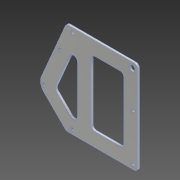
# Autodesk Inventor part: palmrest-plate
Saved by Autodesk Inventor 2018 (Build 220112000, 112)
## iProperties
Created: 2018-07-10
Part Number: palmrest-plate
Material: アルミニウム 6061
Document SubType Name: Sheet Metal
Designer: NaMACHAN
Mass: 31.1777 g
Surface Area: 131.125 cm^2
Volume: 11.5473 cm^3
Density: 2.7 g/cm^3
Sheet Metal Rule: Default
Appearance: アルミニウム - フラット
Flat Pattern Width: 10.477 cm
Flat Pattern Length: 10 cm
Flat Pattern Area: 104.77 cm^2
Sheet Metal Width: 104.770 mm
Sheet Metal Length: 100.000 mm
Sheet Metal Area: 10476.990 mm^2
Author: NaMACHAN
Autodesk Inventor part; units mm, degrees
ref_plane "YZ Plane" through (0, 0, 0) normal (1, 0, 0) x (0, 1, 0)
ref_plane "XZ Plane" through (0, 0, 0) normal (0, 1, 0) x (-1, 0, 0)
ref_plane "XY Plane" through (0, 0, 0) normal (0, 0, 1) x (1, 0, 0)
sketch "スケッチ4" plane through (0, 0, 0) normal (0, 1, 0) x (-1, 0, 0)
  line L0 (0, 0) -> (0, -100)
  line L1 (0, -100) -> (77, -100)
  line L2 (77, -100) -> (107, -70)
  line L3 (107, -70) -> (77, 0)
  line L4 (77, 0) -> (0, 0)
  line L5 (89.2124, -66.5744) -> (70.7868, -85)
  line L6 (65, -85) -> (65, -15)
  line L7 (67.1091, -15) -> (89.2124, -66.5744)
  line L8 (50, -85) -> (50, -15)
  line L9 (50, -15) -> (15, -15)
  line L10 (15, -15) -> (15, -85)
  line L11 (15, -85) -> (50, -85)
  line L12 (70.7868, -85) -> (65, -85)
  line L13 (67.1091, -15) -> (65, -15)
  dimension "d21" = 77
  dimension "d22" = 100
  dimension "d24" = 30
  dimension "d25" = 30
  dimension "d52" = 15
  dimension "d54" = 15
  dimension "d55" = 15
  dimension "d56" = 50
  dimension "d57" = 15
  dimension "d58" = 15
  dimension "d59" = 15
  measures "d21" distance of L3.end L0.start
  measures "d22" distance of L0.start L0.end
  measures "d24" horizontal distance of L1.end L2.end
  measures "d25" horizontal distance of L3.end L2.end
  measures "d52" distance between parallel lines of L0 L10
  measures "d54" distance between parallel lines of L4 L9
  measures "d55" distance between parallel lines of L1 L11
  measures "d56" distance between parallel lines of L0 L8
  measures "d57" distance between parallel lines of L8 L6
  measures "d58" distance between parallel lines of L3 L7
  measures "d59" distance between parallel lines of L2 L5
extrude "プレート2" add sketch "スケッチ4" along normal blind 2
fillet "コーナーR3" radius 12 1 edges at (-107, 1, -70)
fillet "コーナーR4" radius 4 4 edges at (-77, 1, -100) (0, 1, -100) (0, 1, 0) (-77, 1, 0)
sketch "スケッチ5" plane through (0, 2, 0) normal (0, 1, 0) x (1, 0, 0)
  line L0 (-4, 0) -> (-74.3624, 0) projected
  line L1 (0, 96) -> (0, 4) projected
  line L2 (-75.3431, 100) -> (-4, 100) projected
  point P0 (0, 0)
  point P1 (-70, 5)
  point P2 (-70, 95)
  point P3 (-5, 95)
  point P4 (-5, 5)
  point P5 (-5, 45)
  dimension "d29" = 5
  dimension "d30" = 5
  dimension "d31" = 5
  dimension "d40" = 65
  dimension "d73" = 40
  constraints: 3 vertical alignment, 2 horizontal alignment
  measures "d29" distance from line of point (-70, 5) L0
  measures "d30" distance from line of L1 point (-5, 5)
  measures "d31" distance from line of L2 point (-5, 95)
  measures "d40" distance of point (-5, 95) point (-70, 95)
  measures "d73" distance of point (-5, 45) point (-5, 5)
hole "穴2" at (-70, 2, -5) at (-70, 2, -95) at (-5, 2, -95) at (-5, 2, -45) direction (0, -1, 0) diameter 3 end through all
sketch "スケッチ6" plane through (0, 0, 0) normal (0, -1, 0) x (1, 0, 0)
  line L0 (-103.7996, -62.5325) -> (-78.039, -2.4243) projected
  line L1 (-78.1716, -98.8284) -> (-101.2552, -75.7448) projected
  point P0 (0, 0)
  point P1 (-101.0708, -68.8581)
  point P2 (-83.3444, -27.4966)
  dimension "d41" = 5
  dimension "d42" = 5
  dimension "d43" = 5
  dimension "d44" = 45
  measures "d41" distance from line of L0 point (-83.344, -27.497)
  measures "d42" distance from line of L0 point (-101.071, -68.858)
  measures "d43" distance from line of L1 point (-101.071, -68.858)
  measures "d44" distance of point (-101.071, -68.858) point (-83.344, -27.497)
hole "穴3" at (-101.0708, 0, -68.8581) at (-83.3444, 0, -27.4966) direction (0, 1, 0) diameter 3 end through all
fillet "コーナーR5" radius 4 9 edges at (-70.7868, 1, -85) (-65, 1, -85) (-89.2124, 1, -66.5744) (-67.1091, 1, -15) (-65, 1, -15) (-50, 1, -85) (-15, 1, -85) (-50, 1, -15) (-15, 1, -15)
sketch "スケッチ8" plane through (0, 2, 0) normal (0, 1, 0) x (1, 0, 0)
  line L0 (0, 96) -> (0, 4) projected
  line L1 (-4, 0) -> (-74.3624, 0) projected
  point P0 (0, 0)
  point P1 (-6, 6)
  dimension "d74" = 6
  dimension "d75" = 6
  measures "d74" distance from line of L0 point (-6, 6)
  measures "d75" distance from line of L1 point (-6, 6)
hole "穴4" at (-6, 2, -6) direction (0, -1, 0) diameter 6 end through all
equation "\"d38\" = Thickness"
equation "\"d50\" = Thickness"
equation "\"d81\" = Thickness"
equation "\"d26\" = Thickness"
equation "\"BendRadius\" = Thickness"
equation "\"BendReliefWidth\" = Thickness"
equation "\"BendReliefDepth\" = 0.5 * Thickness"
equation "\"CornerReliefSize\" = 4 * Thickness"
equation "\"MinimumRemnant\" = 2 * Thickness"
equation "\"TransitionRadius\" = BendRadius"
equation "\"JacobiRadiusSize\" = Thickness"
equation "\"GapSize\" = Thickness"
equation "\"Thickness\" = 2"
